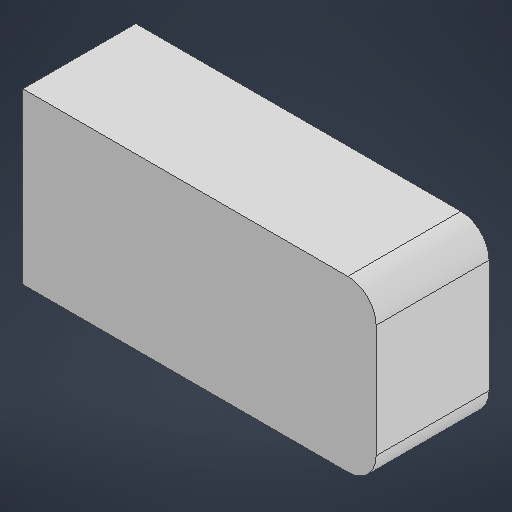
# Autodesk Inventor part: P_Case
Saved by Autodesk Inventor 2026.2 (Build 302298000, 298)
## iProperties
Created: 2025-09-05
Part Number: P_Case
Material: Generisch
Document SubType Name: Modeling
Designer: FAL
Density: 1 g/cm^3
Appearance: Vorgabe
Mass: 1.16843 g
Surface Area: 17.0683 cm^2
Volume: 1.16843 cm^3
Author: FAL
Autodesk Inventor part; units mm, degrees
ref_plane "YZ Plane" through (0, 0, 0) normal (1, 0, 0) x (0, 1, 0)
ref_plane "XZ Plane" through (0, 0, 0) normal (0, 1, 0) x (-1, 0, 0)
ref_plane "XY Plane" through (0, 0, 0) normal (0, 0, 1) x (1, 0, 0)
sketch "Skizze1" plane through (0, 0, 0) normal (0, 1, 0) x (-1, 0, 0)
  line L0 (12.5, 6) -> (-12.5, 6)
  line L1 (-12.5, 6) -> (-12.5, -6)
  line L2 (-12.5, -6) -> (12.5, -6)
  line L3 (12.5, -6) -> (12.5, 6)
  line L4 (12.5, 6) -> (-12.5, -6) construction
  line L5 (-12.5, 6) -> (12.5, -6) construction
  point P0 (0, 0)
  dimension "d0" = 12
  dimension "d2" = 25
  constraints: 12 end point, 2 midpoint, 2 parallel, 1 horizontal, 1 perpendicular
  measures "d0" distance between parallel lines of L2 L0
  measures "d2" distance between parallel lines of L3 L1
extrude "Extrusion1" add sketch "Skizze1" along normal blind 8
fillet "Rundung1" radius 2 2 edges at (12.5, 4, 6) (12.5, 4, -6)
shell "Wandung1" thickness 1.25 removed faces 2 at (-12.5, 2.6667, -2) at (2.8333, 8, -2)
